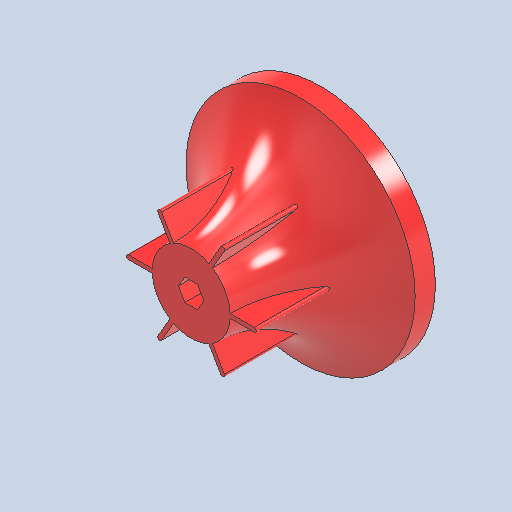
# Autodesk Inventor part: Custom Intake Wheel
Saved by Autodesk Inventor 2022 (Build 260153000, 153)
## iProperties
Created: 2022-09-17
Part Number: Custom Intake Wheel
Material: Generic
Document SubType Name: Modeling
Designer: matt
Density: 1 g/cm^3
Appearance: Default
Author: matt
Autodesk Inventor part; units mm, degrees
ref_plane "YZ Plane" through (0, 0, 0) normal (1, 0, 0) x (0, 1, 0)
ref_plane "XZ Plane" through (0, 0, 0) normal (0, 1, 0) x (-1, 0, 0)
sketch "Sketch1" plane through (0, 0, 0) normal (0, 0, 1) x (1, 0, 0)
  circle A0 centre (0, 0) radius 38.1
  point P0 (0, 38.1)
  dimension "d0" = 76.2
  constraints: 1 coincident, 1 vertical alignment, 2 other
ref_plane "Work Plane1" through (0, 38.1, 0) normal (-1, 0, 0) x (0, -1, 0)
sketch "Sketch2" plane through (0, 38.1, 0) normal (-1, 0, 0) x (0, -1, 0)
  arc A0 (10.0951, -26.7263) -> (28.575, 0) centre (0, 0.0061) ccw
  line L0 (10.1064, 31.68) -> (38.1, 31.68)
  line L1 (38.1, 31.68) -> (38.1, 0)
  line L2 (38.1, -31.68) -> (10.0951, -31.68)
  line L3 (10.0951, -31.68) -> (10.0951, -26.7263)
  line L4 (28.575, 0) -> (38.1, 0)
  line L5 (38.1, 0) -> (38.1, -31.68)
  dimension "d1" = 57.15
  dimension "d2" = 63.36
  constraints: 12 end point, 3 parallel, 2 horizontal, 2 perpendicular, 2 point on circle, 1 centre point, 1 collinear
  measures "d1" diameter of A0
  measures "d2" distance of L0.end L2.start
sweep "Sweep1" add profiles "Sketch2" path "Sketch1"
sketch "Sketch3" plane through (0, 0, 0) normal (0, 0, 1) x (1, 0, 0)
  arc A0 (-5.1836, 7.991) -> (-9.5122, -0.4937) centre (0, 0) ccw
  line L0 (-9.5122, -0.4937) -> (-15.375, -0.4937)
  line L1 (-15.875, 0.0063) -> (-15.875, 0.0063)
  line L2 (-15.375, 0.5063) -> (-9.5115, 0.5063)
  arc A1 (-15.875, 0.0063) -> (-15.375, -0.4937) centre (-15.375, 0.0063) ccw
  arc A2 (-15.375, 0.5063) -> (-15.875, 0.0063) centre (-15.375, 0.0063) ccw
  arc A3 (4.3286, 8.4846) -> (4.3173, 8.4904) centre (0, 0) ccw
  arc A4 (-4.3173, 8.4904) -> (-5.1836, 7.991) centre (0, 0) ccw
  arc A5 (4.3173, 8.4904) -> (-4.3173, 8.4904) centre (0, 0) ccw
  arc A6 (9.5122, 0.4937) -> (5.1942, 7.9841) centre (0, 0) ccw
  arc A7 (5.1942, 7.9841) -> (4.3286, 8.4846) centre (0, 0) ccw
  arc A8 (5.1836, -7.991) -> (9.5115, -0.5063) centre (0, 0) ccw
  arc A9 (9.5115, -0.5063) -> (9.5122, 0.4937) centre (0, 0) ccw
  arc A10 (-4.3286, -8.4846) -> (4.3173, -8.4904) centre (0, 0) ccw
  arc A11 (4.3173, -8.4904) -> (5.1836, -7.991) centre (0, 0) ccw
  arc A12 (-9.5122, -0.4937) -> (-5.1942, -7.9841) centre (0, 0) ccw
  arc A13 (-5.1942, -7.9841) -> (-4.3286, -8.4846) centre (0, 0) ccw
  circle A14 centre (0, 0) radius 9.525 projected
  line L3 (-4.3286, -8.4846) -> (-7.26, -13.562)
  line L4 (-8.126, -13.062) -> (-5.1942, -7.9841)
  arc A15 (-8.126, -13.062) -> (-7.943, -13.745) centre (-7.693, -13.312) ccw
  arc A16 (-7.943, -13.745) -> (-7.26, -13.562) centre (-7.693, -13.312) ccw
  line L5 (5.1836, -7.991) -> (8.115, -13.0683)
  line L6 (7.249, -13.5683) -> (4.3173, -8.4904)
  arc A17 (7.249, -13.5683) -> (7.932, -13.7513) centre (7.682, -13.3183) ccw
  arc A18 (7.932, -13.7513) -> (8.115, -13.0683) centre (7.682, -13.3183) ccw
  line L7 (9.5122, 0.4937) -> (15.375, 0.4937)
  line L8 (15.375, -0.5063) -> (9.5115, -0.5063)
  arc A19 (15.375, -0.5063) -> (15.875, -0.0063) centre (15.375, -0.0063) ccw
  arc A20 (15.875, -0.0063) -> (15.375, 0.4937) centre (15.375, -0.0063) ccw
  line L9 (4.3286, 8.4846) -> (7.26, 13.562)
  line L10 (8.126, 13.062) -> (5.1942, 7.9841)
  arc A21 (8.126, 13.062) -> (7.943, 13.745) centre (7.693, 13.312) ccw
  arc A22 (7.943, 13.745) -> (7.26, 13.562) centre (7.693, 13.312) ccw
  line L11 (-5.1836, 7.991) -> (-8.115, 13.0683)
  line L12 (-7.249, 13.5683) -> (-4.3173, 8.4904)
  arc A23 (-7.249, 13.5683) -> (-7.932, 13.7513) centre (-7.682, 13.3183) ccw
  arc A24 (-7.932, 13.7513) -> (-8.115, 13.0683) centre (-7.682, 13.3183) ccw
  line L13 (-3.1177, -0.0046) -> (-1.5628, 2.6977)
  line L14 (-1.5628, 2.6977) -> (1.5549, 2.7023)
  line L15 (1.5549, 2.7023) -> (3.1177, 0.0046)
  line L16 (3.1177, 0.0046) -> (1.5628, -2.6977)
  line L17 (1.5628, -2.6977) -> (-1.5549, -2.7023)
  line L18 (-1.5549, -2.7023) -> (-3.1177, -0.0046)
  point P0 (-15.875, 0.5063)
  point P1 (-15.875, -0.4937)
  point P2 (-7.51, -13.995)
  point P3 (-8.376, -13.495)
  point P4 (8.365, -13.5013)
  point P5 (7.499, -14.0013)
  point P6 (15.875, 0.4937)
  point P7 (15.875, -0.5063)
  point P8 (7.51, 13.995)
  point P9 (8.376, 13.495)
  point P10 (-8.365, 13.5013)
  point P11 (-7.499, 14.0013)
  point P12 (-7.943, -13.745)
  point P13 (-4.3286, -8.4846)
  point P14 (-5.1942, -7.9841)
  point P15 (15.875, -0.0063)
  point P16 (9.5122, 0.4937)
  point P17 (9.5115, -0.5063)
  point P18 (7.943, 13.745)
  point P19 (4.3286, 8.4846)
  point P20 (5.1942, 7.9841)
  point P21 (-5.1836, 7.991)
  dimension "d5" = 1
  dimension "d6" = 0.5
  dimension "d13" = 360
  dimension "d17" = 5.4
  constraints: 51 point on circle, 38 end point, 24 centre point, 14 point on line, 4 tangent, 1 coincident, 1 concentric, 1 horizontal, 1 parallel, 1 perpendicular, 100 other
  measures "d5" distance of point (-15.875, -0.494) point (-15.875, 0.506)
  measures "d6" radius of A1
  measures "d17" distance between parallel lines of L17 L14
extrude "Extrusion1" add sketch "Sketch3" against normal up to surface contours L11 A24 A23 L12 A4 | A0 L0 A1 A2 L2 | A13 L3 A16 A15 L4 | L9 A22 A21 L10 A7 | A11 L5 A18 A17 L6 | L7 A20 A19 L8 A9
extrude "Extrusion2" cut sketch "Sketch3" against normal through all contours L13 L14 L15 L16 L17 L18
body "Solid1"
